Autodesk Inventor part; units mm, degrees
(part 2 of 2)
  arc A291 (24.8565, 31.8046) -> (23.8053, 31.1147) centre (31.3964, 20.6936) ccw projected
  arc A292 (23.8053, 31.1147) -> (23.1322, 30.5755) centre (29.291, 23.5772) ccw projected
  arc A293 (23.1322, 30.5755) -> (21.9307, 31.4483) centre (0, 0) ccw projected
  arc A294 (21.9307, 31.4483) -> (22.2356, 32.2552) centre (13.3718, 35.1431) ccw projected
  arc A295 (22.2356, 32.2552) -> (22.5669, 33.4681) centre (9.9788, 36.2544) ccw projected
  arc A296 (22.5669, 33.4681) -> (22.8546, 35.1883) centre (6.2739, 37.0778) ccw projected
  arc A297 (22.8546, 35.1883) -> (20.9772, 36.3388) centre (0, 0) ccw projected
  arc A298 (20.9772, 36.3388) -> (19.5752, 35.3014) centre (30.1882, 22.4231) ccw projected
  arc A299 (19.5752, 35.3014) -> (18.6448, 34.4556) centre (27.7726, 25.3503) ccw projected
  arc A300 (18.6448, 34.4556) -> (18.0643, 33.8177) centre (25.2421, 27.869) ccw projected
  arc A301 (18.0643, 33.8177) -> (16.7411, 34.4919) centre (0, 0) ccw projected
  arc A302 (16.7411, 34.4919) -> (16.916, 35.3365) centre (7.7096, 36.8023) ccw projected
  arc A303 (16.916, 35.3365) -> (17.0535, 36.5863) centre (4.1845, 37.3691) ccw projected
  arc A304 (17.0535, 36.5863) -> (17.0686, 38.3303) centre (0.3965, 37.6027) ccw projected
  arc A305 (17.0686, 38.3303) -> (15.0343, 39.1729) centre (0, 0) ccw projected
  arc A306 (15.0343, 39.1729) -> (13.8118, 37.9291) centre (26.3088, 26.8695) ccw projected
  arc A307 (13.8118, 37.9291) -> (13.0252, 36.9481) centre (23.4651, 29.3828) ccw projected
  arc A308 (13.0252, 36.9481) -> (12.5517, 36.2272) centre (20.5717, 31.4746) ccw projected
  arc A309 (12.5517, 36.2272) -> (11.1393, 36.6861) centre (0, 0) ccw projected
  arc A310 (11.1393, 36.6861) -> (11.1799, 37.5477) centre (1.8575, 37.5552) ccw projected
  arc A311 (11.1799, 37.5477) -> (11.1201, 38.8036) centre (-1.7129, 37.5636) ccw projected
  arc A312 (11.1201, 38.8036) -> (10.8623, 40.5285) centre (-5.4908, 37.2018) ccw projected
  arc A313 (10.8623, 40.5285) -> (8.7212, 41.0425) centre (0, 0) ccw projected
  arc A314 (8.7212, 41.0425) -> (7.7084, 39.6227) centre (21.7816, 30.6543) ccw projected
  arc A315 (7.7084, 39.6227) -> (7.0849, 38.5308) centre (18.5797, 32.6918) ccw projected
  arc A316 (7.0849, 38.5308) -> (6.73, 37.7447) centre (15.3947, 34.3052) ccw projected
  arc A317 (6.73, 37.7447) -> (5.2632, 37.977) centre (0, 0) ccw projected
  arc A318 (5.2632, 37.977) -> (5.1685, 38.8343) centre (-4.0403, 37.3834) ccw projected
  arc A319 (5.1685, 38.8343) -> (4.9158, 40.0547) centre (-7.568, 36.8332) ccw projected
  arc A320 (4.9158, 40.0547) -> (4.3885, 41.7288) centre (-11.2428, 35.8848) ccw projected
  arc A321 (4.3885, 41.7288) -> (2.1934, 41.9015) centre (0, 0) ccw projected
  arc A322 (2.1934, 41.9015) -> (1.4107, 40.3306) centre (16.718, 33.6843) ccw projected
  arc A323 (1.4107, 40.3306) -> (0.9701, 39.1647) centre (13.2368, 35.1958) ccw projected
  arc A324 (0.9701, 39.1647) -> (0.7425, 38.3328) centre (9.8386, 36.2911) ccw projected
  circle A325 centre (48.0782, 6.3084) radius 1.5
  circle A326 centre (48.4833, 0.8234) radius 1.5
  circle A327 centre (53.031, 3.9168) radius 1.5
  circle A328 centre (49.8642, 3.6829) radius 4.6754
  circle A329 centre (49.8642, 3.6829) radius 9.6754
  line L1 (0, 0) -> (49.8642, 3.6829)
  line L2 (0, 0) -> (10.1914, 20.9974)
  line L3 (0, 0) -> (-3.204, -23.119)
  arc A330 (10.1914, 20.9974) -> (14.6249, 13.8146) centre (14.6896, 18.8142) ccw
  arc A331 (0.5067, -18.9621) -> (-3.204, -23.119) centre (1.7486, -23.8054) ccw
  line L4 (14.6249, 13.8146) -> (49.9892, 13.3575)
  line L5 (0.5067, -18.9621) -> (52.2675, -5.6893)
  line L6 (10.1914, 20.9974) -> (16.7411, 34.4919)
  line L7 (-3.204, -23.119) -> (-5.2632, -37.977)
  point P0 (37.977, 5.2632)
  point P1 (37.7447, 6.73)
  point P2 (4.3665, 8.9963)
  point P3 (-16.7411, 34.4919)
  point P4 (-18.0643, 33.8177)
  point P5 (-1.3728, -9.9053)
  point P6 (37.585, 13.5178)
  point P7 (40.8953, -8.6054)
  point P8 (40.2608, 4.8612)
  point P9 (40.4471, 1.4618)
  dimension "d2" = 6
  dimension "d3" = 6.13
  dimension "d5" = 7
  dimension "d74" = 5
  dimension "d79" = 5
  dimension "d80" = 5
  dimension "d81" = 15
  dimension "d82" = 15
  constraints: 16 end point, 11 tangent, 10 centre point, 9 point on circle, 2 coincident, 2 point on line, 1 vertical, 6 other
  measures "d2" diameter of A0
  measures "d3" radial gap between concentric circles of A1 A2
  measures "d5" radial gap between concentric circles of A0 A3
  measures "d74" radial gap between concentric circles of A328 A329
  measures "d79" radius of A330
  measures "d80" radius of A331
  measures "d81" distance of L2.end L6.end
  measures "d82" distance of L3.end L7.end
extrude "押し出し6" cut sketch "Sketch2" against normal blind 8 contours A0 L3 L1 | L1 L2 A0 | A0 L2 L3 | A331 L5 A1 L7 | L6 A1 L4 A330 | A1 L6 A301 A300 A299 A298 A297 A296 A295 A294 A293 A292 A291 A290 A289 A288 A287 A286 A285 A284 A283 A282 A281 A280 A279 A278 A277 A276 A275 A274 A273 A272 A271 A270 A269 A268 A267 A266 A265 A264 A263 L4 | L1 A249 A248 A329 | A329 A250 A249 L1 | A1 L5 A234 A233 A232 A231 A230 A229 A228 A227 A226 A225 A224 A223 A222 A221 A220 A219 A218 A217 A216 A215 A214 A213 A212 A211 A210 A209 A208 A207 A206 A205 A204 A203 A202 A201 A200 A199 A198 A197 A196 A195 A194 A193 A192 A191 A190 A189 A188 A187 A186 A185 A184 A183 A182 A181 A180 A179 A178 A177 A176 A175 A174 A173 A172 A171 A170 A169 A168 A167 A166 A165 A164 A163 A162 A161 A160 A159 A158 L7 | L4 A329 A250 A251 A252 A4 A254 A255 A256 A257 A258 A259 A260 A261 A262 A263 | A328 | A329 A248 A249 A250 | A329 L5 A234 A235 A236 A237 A238 A239 A240 A241 A242 A243 A244 A245 A246 A247 A248
extrude "押し出し10" add sketch "Sketch2" against normal blind 8 contours L1 A249 A248 A329 | A329 A250 A249 L1 | L4 A329 A250 A251 A252 A4 A254 A255 A256 A257 A258 A259 A260 A261 A262 A263 | A328 | A329 A248 A249 A250 | A329 L5 A234 A235 A236 A237 A238 A239 A240 A241 A242 A243 A244 A245 A246 A247 A248
sketch "スケッチ7" plane through (0, 0, 0) normal (0, 0, 1) x (1, 0, 0)
  circle A0 centre (48.4833, 0.8234) radius 1.5 projected
  circle A1 centre (53.031, 3.9168) radius 1.5 projected
  circle A2 centre (48.0782, 6.3084) radius 1.5 projected
  circle A3 centre (48.4833, 0.8234) radius 3
  circle A4 centre (48.0782, 6.3084) radius 3
  circle A5 centre (53.031, 3.9168) radius 3
  point P0 (0, 0)
  point P1 (47.0851, 3.4776)
  point P2 (51.4315, 1.3787)
  point P3 (51.076, 6.1923)
  dimension "d85" = 6
  dimension "d86" = 6
  dimension "d87" = 6
  constraints: 3 centre point, 3 coincident
  measures "d85" diameter of A3
  measures "d86" diameter of A4
  measures "d87" diameter of A5
extrude "押し出し11" cut sketch "スケッチ7" against normal blind 3
sketch "スケッチ9" plane through (0, 0, -8) normal (0, 0, -1) x (-1, 0, 0)
  point P0 (0, 0)
body "Solid1"
